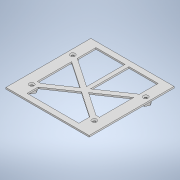
# Autodesk Inventor part: top_base
Saved by Autodesk Inventor 2020.2 (Build 242310000, 310)
## iProperties
Created: 2021-09-14
Part Number: top_base
Material: Generic
Document SubType Name: Modeling
Designer: Tarsoly
Density: 1 g/cm^3
Appearance: Default
Author: Tarsoly
Autodesk Inventor part; units mm, degrees
ref_plane "YZ Plane" through (0, 0, 0) normal (1, 0, 0) x (0, 1, 0)
ref_plane "XZ Plane" through (0, 0, 0) normal (0, 1, 0) x (-1, 0, 0)
ref_plane "XY Plane" through (0, 0, 0) normal (0, 0, 1) x (1, 0, 0)
sketch "Sketch1" plane through (0, 0, 0) normal (0, 1, 0) x (-1, 0, 0)
  circle A0 centre (0, 0) radius 80 construction
  line L0 (56.002, 57.1295) -> (-56.002, 57.1295) construction
  line L1 (-56.002, 57.1295) -> (-56.002, -57.1295) construction
  line L2 (-56.002, -57.1295) -> (56.002, -57.1295) construction
  line L3 (56.002, -57.1295) -> (56.002, 57.1295) construction
  line L4 (56.002, 57.1295) -> (-56.002, -57.1295) construction
  line L5 (-56.002, 57.1295) -> (56.002, -57.1295) construction
  line L6 (54.002, 55.1295) -> (-54.002, 55.1295)
  line L7 (-54.002, 55.1295) -> (-54.002, -55.1295)
  line L8 (-54.002, -55.1295) -> (54.002, -55.1295)
  line L9 (54.002, -55.1295) -> (54.002, 55.1295)
  dimension "d0" = 160
  dimension "d1" = 2
  constraints: 20 end point, 4 parallel, 2 midpoint, 2 perpendicular, 1 coincident, 1 horizontal, 6 other
  measures "d1" distance between parallel lines of L3 L9
extrude "Extrusion1" add sketch "Sketch1" along normal blind 2
sketch "Sketch2" plane through (0, 0, 0) normal (0, -1, 0) x (1, 0, 0)
  line L0 (-39.0523, 32.251) -> (-42.2277, 32.251) construction
  line L1 (-42.2277, 32.251) -> (-43.8154, 35.001) construction
  line L2 (-43.8154, 35.001) -> (-42.2277, 37.751) construction
  line L3 (-42.2277, 37.751) -> (-39.0523, 37.751) construction
  line L4 (-39.0523, 37.751) -> (-37.4646, 35.001) construction
  line L5 (-37.4646, 35.001) -> (-39.0523, 32.251) construction
  line L6 (42.2277, 32.251) -> (39.0523, 32.251) construction
  line L7 (39.0523, 32.251) -> (37.4646, 35.001) construction
  line L8 (37.4646, 35.001) -> (39.0523, 37.751) construction
  line L9 (39.0523, 37.751) -> (42.2277, 37.751) construction
  line L10 (42.2277, 37.751) -> (43.8154, 35.001) construction
  line L11 (43.8154, 35.001) -> (42.2277, 32.251) construction
  line L12 (48.9587, -27.749) -> (45.7833, -27.749) construction
  line L13 (45.7833, -27.749) -> (44.1956, -24.999) construction
  line L14 (44.1956, -24.999) -> (45.7833, -22.249) construction
  line L15 (45.7833, -22.249) -> (48.9587, -22.249) construction
  line L16 (48.9587, -22.249) -> (50.5464, -24.999) construction
  line L17 (50.5464, -24.999) -> (48.9587, -27.749) construction
  line L18 (-45.7833, -22.249) -> (-44.1956, -24.999) construction
  line L19 (-44.1956, -24.999) -> (-45.7833, -27.749) construction
  line L20 (-45.7833, -27.749) -> (-48.9587, -27.749) construction
  line L21 (-48.9587, -27.749) -> (-50.5464, -24.999) construction
  line L22 (-50.5464, -24.999) -> (-48.9587, -22.249) construction
  line L23 (-48.9587, -22.249) -> (-45.7833, -22.249) construction
  line L24 (-47.371, -24.999) -> (47.371, -24.999) construction
  line L25 (-40.64, 35.001) -> (40.64, 35.001) construction
  line L26 (-75.6027, 0) -> (75.6027, 0) construction
  line L27 (0, -77.1813) -> (0, 77.1813) construction
  line L28 (-37.3491, 35.001) -> (-38.9946, 37.851)
  line L29 (-38.9946, 37.851) -> (-42.2854, 37.851)
  line L30 (-42.2854, 37.851) -> (-43.9309, 35.001)
  line L31 (-43.9309, 35.001) -> (-42.2854, 32.151)
  line L32 (-42.2854, 32.151) -> (-38.9946, 32.151)
  line L33 (-38.9946, 32.151) -> (-37.3491, 35.001)
  line L34 (49.0164, -27.849) -> (45.7256, -27.849)
  line L35 (45.7256, -27.849) -> (44.0801, -24.999)
  line L36 (44.0801, -24.999) -> (45.7256, -22.149)
  line L37 (45.7256, -22.149) -> (49.0164, -22.149)
  line L38 (49.0164, -22.149) -> (50.6619, -24.999)
  line L39 (50.6619, -24.999) -> (49.0164, -27.849)
  line L40 (43.9309, 35.001) -> (42.2854, 37.851)
  line L41 (42.2854, 37.851) -> (38.9946, 37.851)
  line L42 (38.9946, 37.851) -> (37.3491, 35.001)
  line L43 (37.3491, 35.001) -> (38.9946, 32.151)
  line L44 (38.9946, 32.151) -> (42.2854, 32.151)
  line L45 (42.2854, 32.151) -> (43.9309, 35.001)
  line L46 (-45.7256, -27.849) -> (-44.0801, -24.999)
  line L47 (-44.0801, -24.999) -> (-45.7256, -22.149)
  line L48 (-45.7256, -22.149) -> (-49.0164, -22.149)
  line L49 (-49.0164, -22.149) -> (-50.6619, -24.999)
  line L50 (-50.6619, -24.999) -> (-49.0164, -27.849)
  line L51 (-49.0164, -27.849) -> (-45.7256, -27.849)
  line L52 (-35.0397, 35.001) -> (-37.8399, 39.851)
  line L53 (-37.8399, 39.851) -> (-43.4401, 39.851)
  line L54 (-43.4401, 39.851) -> (-46.2403, 35.001)
  line L55 (-46.2403, 35.001) -> (-43.4401, 30.151)
  line L56 (-43.4401, 30.151) -> (-37.8399, 30.151)
  line L57 (-37.8399, 30.151) -> (-35.0397, 35.001)
  line L58 (46.2403, 35.001) -> (43.4401, 39.851)
  line L59 (43.4401, 39.851) -> (37.8399, 39.851)
  line L60 (37.8399, 39.851) -> (35.0397, 35.001)
  line L61 (35.0397, 35.001) -> (37.8399, 30.151)
  line L62 (37.8399, 30.151) -> (43.4401, 30.151)
  line L63 (43.4401, 30.151) -> (46.2403, 35.001)
  line L64 (44.5709, -29.849) -> (50.1711, -29.849)
  line L65 (50.1711, -29.849) -> (52.9713, -24.999)
  line L66 (52.9713, -24.999) -> (50.1711, -20.149)
  line L67 (50.1711, -20.149) -> (44.5709, -20.149)
  line L68 (44.5709, -20.149) -> (41.7707, -24.999)
  line L69 (41.7707, -24.999) -> (44.5709, -29.849)
  line L70 (-44.5709, -29.849) -> (-41.7707, -24.999)
  line L71 (-41.7707, -24.999) -> (-44.5709, -20.149)
  line L72 (-44.5709, -20.149) -> (-50.1711, -20.149)
  line L73 (-50.1711, -20.149) -> (-52.9713, -24.999)
  line L74 (-52.9713, -24.999) -> (-50.1711, -29.849)
  line L75 (-50.1711, -29.849) -> (-44.5709, -29.849)
  point P0 (0, 0)
  point P1 (0, 35.001)
  point P2 (0, -24.999)
  dimension "d4" = 5.5
  dimension "d5" = 5.5
  dimension "d6" = 5.5
  dimension "d7" = 5.5
  dimension "d8" = 81.28
  dimension "d9" = 94.742
  dimension "d10" = 24.999
  dimension "d11" = 35.001
  dimension "d12" = 0.1
  dimension "d13" = 0.1
  dimension "d14" = 0.1
  dimension "d15" = 0.1
  dimension "d16" = 2
  dimension "d17" = 2
  dimension "d18" = 2
  dimension "d19" = 2
  constraints: 148 end point, 5 horizontal, 3 point on line, 2 midpoint, 92 other
  measures "d4" distance between parallel lines of L4 L1
  measures "d5" distance between parallel lines of L10 L7
  measures "d6" distance between parallel lines of L16 L13
  measures "d7" distance between parallel lines of L22 L19
  measures "d8" distance of L25.end L25.start
  measures "d9" distance of L24.start L24.end
  measures "d10" distance between parallel lines of L26 L24
  measures "d11" distance between parallel lines of L26 L25
  measures "d12" distance between parallel lines of L4 L28
  measures "d13" distance between parallel lines of L17 L39
  measures "d14" distance between parallel lines of L10 L40
  measures "d15" distance between parallel lines of L19 L46
  measures "d16" distance between parallel lines of L33 L57
  measures "d17" distance between parallel lines of L45 L63
  measures "d18" distance between parallel lines of L34 L64
  measures "d19" distance between parallel lines of L51 L75
extrude "Extrusion2" add sketch "Sketch2" along normal blind 5
sketch "Sketch3" plane through (0, 2, 0) normal (0, 1, 0) x (1, 0, 0)
  line L0 (-42.2854, -37.851) -> (-43.9309, -35.001) construction
  line L1 (-43.9309, -35.001) -> (-42.2854, -32.151) construction
  line L2 (-42.2854, -32.151) -> (-38.9946, -32.151) construction
  line L3 (-38.9946, -32.151) -> (-37.3491, -35.001) construction
  line L4 (-37.3491, -35.001) -> (-38.9946, -37.851) construction
  line L5 (-38.9946, -37.851) -> (-42.2854, -37.851) construction
  line L6 (-50.6619, 24.999) -> (-49.0164, 27.849) construction
  line L7 (-49.0164, 27.849) -> (-45.7256, 27.849) construction
  line L8 (-45.7256, 27.849) -> (-44.0801, 24.999) construction
  line L9 (-44.0801, 24.999) -> (-45.7256, 22.149) construction
  line L10 (-45.7256, 22.149) -> (-49.0164, 22.149) construction
  line L11 (-49.0164, 22.149) -> (-50.6619, 24.999) construction
  line L12 (50.6619, 24.999) -> (49.0164, 22.149) construction
  line L13 (49.0164, 22.149) -> (45.7256, 22.149) construction
  line L14 (45.7256, 22.149) -> (44.0801, 24.999) construction
  line L15 (44.0801, 24.999) -> (45.7256, 27.849) construction
  line L16 (45.7256, 27.849) -> (49.0164, 27.849) construction
  line L17 (49.0164, 27.849) -> (50.6619, 24.999) construction
  line L18 (42.2854, -32.151) -> (43.9309, -35.001) construction
  line L19 (43.9309, -35.001) -> (42.2854, -37.851) construction
  line L20 (42.2854, -37.851) -> (38.9946, -37.851) construction
  line L21 (38.9946, -37.851) -> (37.3491, -35.001) construction
  line L22 (37.3491, -35.001) -> (38.9946, -32.151) construction
  line L23 (38.9946, -32.151) -> (42.2854, -32.151) construction
  line L24 (47.371, 27.849) -> (47.371, 22.149) construction
  line L25 (49.0164, 22.149) -> (50.6619, 24.999) construction
  line L26 (-49.0164, 22.149) -> (-50.6619, 24.999) construction
  line L27 (50.6619, 24.999) -> (-50.6619, 24.999) construction
  line L28 (-49.0164, 27.849) -> (-45.7256, 27.849) construction
  line L29 (-47.371, 27.849) -> (-47.371, 22.149) construction
  line L30 (-45.7256, 22.149) -> (-49.0164, 22.149) construction
  line L31 (-38.9946, -37.851) -> (-42.2854, -37.851) construction
  line L32 (-40.64, -37.851) -> (-40.64, -32.151) construction
  line L33 (-43.9309, -35.001) -> (43.9309, -35.001) construction
  line L34 (38.9946, -32.151) -> (42.2854, -32.151) construction
  line L35 (40.64, -32.151) -> (40.64, -37.851) construction
  point P0 (0, 0)
  point P1 (-47.371, 24.999)
  point P2 (47.371, 24.999)
  point P3 (40.64, -35.001)
  point P4 (-40.64, -35.001)
  constraints: 12 end point, 12 midpoint, 2 point on line, 1 horizontal, 1 perpendicular
hole "Hole1" at (-47.371, 2, -24.999) at (47.371, 2, -24.999) at (40.64, 2, 35.001) at (-40.64, 2, 35.001) direction (0, -1, 0) diameter 3.4 end through all countersink diameter 6.3 countersink angle 90 clearance for "Countersunk Flat Head Screw ISO 2009/7046" size "M3" standard "ISO"
sketch "Sketch4" plane through (0, 2, 0) normal (0, 1, 0) x (1, 0, 0)
  line L0 (-40.371, 48.1295) -> (40.371, 48.1295)
  line L1 (40.371, 48.1295) -> (40.371, -28.001)
  line L2 (-40.371, -28.001) -> (-40.371, 48.1295)
  line L3 (33.64, -28.001) -> (33.64, -48.1295)
  line L4 (33.64, -48.1295) -> (-33.64, -48.1295)
  line L5 (-33.64, -48.1295) -> (-33.64, -28.001)
  circle A0 centre (47.371, 24.999) radius 3.15 construction
  circle A1 centre (-47.371, 24.999) radius 3.15 construction
  line L6 (54.002, 55.1295) -> (-54.002, 55.1295) construction
  circle A2 centre (40.64, -35.001) radius 3.15 construction
  circle A3 centre (-40.64, -35.001) radius 3.15 construction
  line L7 (-54.002, -55.1295) -> (54.002, -55.1295) construction
  line L8 (40.371, -28.001) -> (33.64, -28.001)
  line L9 (-33.64, -28.001) -> (-40.371, -28.001)
  circle A4 centre (-47.371, 24.999) radius 1.7 construction
  circle A5 centre (40.64, -35.001) radius 1.7 construction
  line L10 (-47.371, 24.999) -> (40.64, -35.001) construction
  line L11 (47.371, 24.999) -> (-40.64, -35.001) construction
  line L12 (-40.371, 23.8577) -> (35.6979, -28.001)
  line L13 (-40.371, 16.5961) -> (33.64, -33.8597)
  line L14 (40.371, 16.5961) -> (-33.64, -33.8597)
  line L15 (40.371, 23.8577) -> (-35.6979, -28.001)
  line L16 (-2.5, 48.1295) -> (2.5, 48.1295)
  line L17 (2.5, 48.1295) -> (2.5, -1.9602)
  line L18 (2.5, -1.9602) -> (-2.5, -1.9602)
  line L19 (-2.5, -1.9602) -> (-2.5, 48.1295)
  point P0 (0, -10.9262)
  point P1 (5.3259, -7.2954)
  point P2 (-5.3259, -7.2954)
  dimension "d35" = 7
  dimension "d36" = 7
  dimension "d37" = 7
  dimension "d38" = 7
  dimension "d40" = 7
  dimension "d41" = 7
  dimension "d42" = 7
  dimension "d43" = 3
  dimension "d44" = 3
  dimension "d45" = 3
  dimension "d46" = 3
  dimension "d47" = 5
  constraints: 36 end point, 11 point on line, 10 parallel, 3 perpendicular, 2 horizontal, 1 collinear
  measures "d35" distance from line of L11.start L1
  measures "d36" distance from line of A1.centre L2
  measures "d37" distance between parallel lines of L6 L0
  measures "d38" distance from line of A2.centre L3
  measures "d40" distance from line of L11.end L5
  measures "d41" distance between parallel lines of L4 L7
  measures "d42" distance from line of A2.centre L8
  measures "d43" distance between parallel lines of L10 L12
  measures "d44" distance between parallel lines of L10 L13
  measures "d45" distance between parallel lines of L11 L14
  measures "d46" distance between parallel lines of L11 L15
  measures "d47" distance between parallel lines of L17 L19
extrude "Extrusion3" cut sketch "Sketch4" against normal through all contours L0 L19 L12 L2 | L0 L1 L15 L17 | L13 L15 L9 L2 | L14 L1 L8 L12 | L13 L3 L4 L5 L14
equation "\"d5\" = d4"
equation "\"d6\" = d4"
equation "\"d7\" = d4"
equation "\"d17\" = d16"
equation "\"d18\" = d16"
equation "\"d19\" = d16"
equation "\"d36\" = d35"
equation "\"d37\" = d35"
equation "\"d38\" = d35"
equation "\"d40\" = d35"
equation "\"d41\" = d35"
equation "\"d42\" = d35"
equation "\"d44\" = d43"
equation "\"d45\" = d43"
equation "\"d46\" = d43"
equation "\"d39\" = d35"
body "Solid1"
